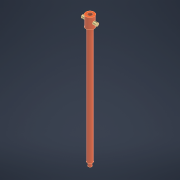
# Autodesk Inventor part: boom 3
Saved by Autodesk Inventor 2021 (Build 250183000, 183)
## iProperties
Created: 2020-12-24
Part Number: boom 3
Material: Steel, Mild
Document SubType Name: Modeling
Designer: Vikki
Density: 7.85 g/cm^3
Appearance: Smooth - Light Orange
Mass: 118.153 g
Surface Area: 81.4016 cm^2
Volume: 15.0513 cm^3
Author: Vikki
Autodesk Inventor part; units mm, degrees
ref_plane "XZ Plane" through (0, 0, 0) normal (0, 1, 0) x (-1, 0, 0)
ref_plane "XY Plane" through (0, 0, 0) normal (0, 0, 1) x (1, 0, 0)
sketch "Sketch1" plane through (0, 0, 0) normal (0, 1, 0) x (-1, 0, 0)
  circle A0 centre (0, 0) radius 5
  dimension "d0" = 10
  constraints: 1 centre point, 1 coincident
  measures "d0" diameter of A0
extrude "Extrusion1" add sketch "Sketch1" along normal blind 240
sketch "Sketch2" plane through (0, 240, 0) normal (0, 1, 0) x (1, 0, 0)
  circle A0 centre (0, 0) radius 4.25
  circle A1 centre (0, 0) radius 7.75
  dimension "d3" = 8.5
  dimension "d4" = 15.5
  constraints: 2 centre point, 2 coincident
  measures "d3" diameter of A0
  measures "d4" diameter of A1
extrude "Extrusion2" add sketch "Sketch2" against normal blind 20
ref_plane "Work Plane1" through (-7.75, 240, 0) normal (1, 0, 0) x (0, 1, 0)
sketch "Sketch3" plane through (-7.75, 240, 0) normal (1, 0, 0) x (0, 1, 0)
  circle A0 centre (-10, 0) radius 3
  line L0 (0, -7.75) -> (0, 7.75) projected
  point P0 (-240, 0)
  point P1 (0, 0)
  dimension "d7" = 6
  dimension "d8" = 10
  constraints: 1 centre point, 1 horizontal alignment, 1 midpoint
  measures "d7" diameter of A0
  measures "d8" distance from line of L0 A0.centre
extrude "Extrusion3" add sketch "Sketch3" along normal blind 2 and the other way blind 6
mirror "Mirror1" about plane through (0, 0, 0) normal (1, 0, 0) of "Extrusion3"
sketch "Sketch4" plane through (0, 0, 0) normal (0, -1, 0) x (1, 0, 0)
  circle A0 centre (0, 0) radius 3.25
  dimension "d13" = 6.5
  constraints: 1 centre point, 1 coincident
  measures "d13" diameter of A0
extrude "Extrusion4" add sketch "Sketch4" along normal blind 7
sketch "Sketch5" plane through (0, 240, 0) normal (0, 1, 0) x (1, 0, 0)
  circle A0 centre (0, 0) radius 7.75 projected
  circle A1 centre (0, 0) radius 4
  dimension "d16" = 8
  constraints: 1 centre point, 1 coincident
  measures "d16" diameter of A1
extrude "Extrusion5" cut sketch "Sketch5" against normal blind 16 contours A1
sketch "Sketch6" plane through (13.75, 230, 0) normal (1, 0, 0) x (0, 0, -1)
  circle A0 centre (0, 0) radius 3 projected
  point P0 (0, -230)
extrude "Extrusion6" add sketch "Sketch6" against normal up to surface (27.5 mm away)
body "Solid1"
